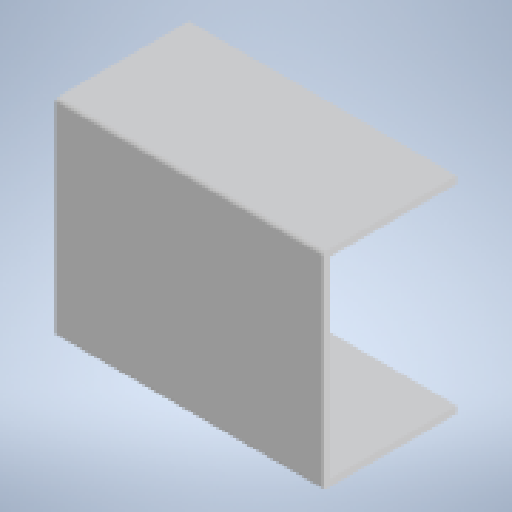
# Autodesk Inventor part: WingBoxCouple
Saved by Autodesk Inventor 2026 (Build 300175050, 175E)
## iProperties
Created: 2025-07-20
Part Number: WingBoxCouple
Material: Generic
Document SubType Name: Modeling
Designer: Cupri
Density: 1 g/cm^3
Appearance: Default
Author: Cupri
Autodesk Inventor part; units mm, degrees
ref_plane "YZ Plane" through (0, 0, 0) normal (1, 0, 0) x (0, 1, 0)
ref_plane "XZ Plane" through (0, 0, 0) normal (0, 1, 0) x (-1, 0, 0)
ref_plane "XY Plane" through (0, 0, 0) normal (0, 0, 1) x (1, 0, 0)
sketch "Sketch14" plane through (0, 0, 0) normal (1, 0, 0) x (0, 1, 0)
  line L0 (0, 4.9685) -> (-195, 4.9685)
  line L1 (-195, 4.9685) -> (-195, -122.0315)
  line L2 (-195, -122.0315) -> (0, -122.0315)
  line L3 (0, -122.0315) -> (0, 4.9685)
  line L4 (-6.35, -1.3815) -> (-188.65, -1.3815)
  line L5 (-188.65, -1.3815) -> (-188.65, -115.6815)
  line L6 (-188.65, -115.6815) -> (-6.35, -115.6815)
  line L7 (-6.35, -115.6815) -> (-6.35, -1.3815)
  line L8 (0, 4.9685) -> (-195, 4.9685)
  point P0 (0, 0)
  constraints: 18 end point
extrude "Extrusion10" add sketch "Sketch14" against normal blind 254
sketch "Sketch18" plane through (-254, 0, 0) normal (-1, 0, 0) x (0, 0, 1)
  line L0 (-1.3815, -188.65) -> (-115.6815, -188.65) projected
  line L1 (-122.0315, 0) -> (-122.0315, -195) projected
  line L2 (-115.6815, -188.65) -> (-122.0315, -188.65)
  line L3 (-122.0315, -188.65) -> (-122.0315, -6.6525)
  line L4 (-122.0315, -6.6525) -> (-115.6815, -6.6525)
  line L5 (-115.6815, -6.6525) -> (-115.6815, -188.65)
  point P0 (0, 0)
  constraints: 8 end point, 2 parallel, 1 horizontal, 1 perpendicular, 1 point on line
extrude "Extrusion14" cut sketch "Sketch18" against normal through all
fillet "Fillet3" radius 3.175 2 edges at (-127, 0, 4.9685) (-127, -195, 4.9685)
body "Solid2"
